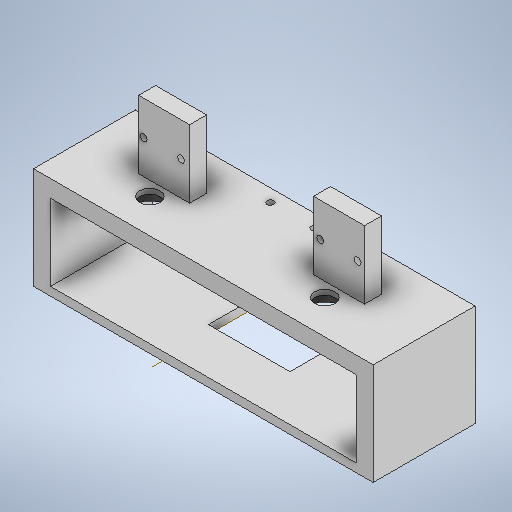
# Autodesk Inventor part: upper part shooter
Saved by Autodesk Inventor 2025.3 (Build 293356000, 356)
## iProperties
Created: 2026-04-10
Part Number: upper part shooter
Material: Generic
Document SubType Name: Modeling
Designer: lenovo
Density: 1 g/cm^3
Appearance: Default
Author: lenovo
## iProperties of the stored document upper part shooter_3DPrint.ipt
Created: 2026-04-14
Part Number: upper part shooter_3DPrint
Material: Generic
Document SubType Name: Modeling
Designer: lenovo
Density: 1 g/cm^3
Appearance: Default
Author: lenovo
Autodesk Inventor part; units mm, degrees
ref_plane "YZ Plane" through (0, 0, 0) normal (1, 0, 0) x (0, 1, 0)
ref_plane "XZ Plane" through (0, 0, 0) normal (0, 1, 0) x (-1, 0, 0)
ref_plane "XY Plane" through (0, 0, 0) normal (0, 0, 1) x (1, 0, 0)
sketch "Sketch1" plane through (0, 0, 0) normal (0, 1, 0) x (-1, 0, 0)
  line L0 (0, -35) -> (4, -35)
  line L1 (-48, 0) -> (-48, -35)
  line L2 (-48, -24.7754) -> (-48, -13.3333)
  line L3 (-48, -35) -> (-52, -35)
  line L4 (-52, -35) -> (-52, -33)
  line L5 (-52, -33) -> (-124, -33)
  line L6 (4, -35) -> (4, -33)
  line L7 (4, -33) -> (76, -33)
  line L8 (0, 0) -> (0, -35)
  line L9 (0, -96.6) -> (0, 47.6) projected
  line L10 (0, 0) -> (-48, 0)
  line L11 (76, -33) -> (76, 27)
  line L12 (76, 27) -> (-124, 27)
  line L13 (-124, 27) -> (-124, -33)
  line L14 (-24, 27) -> (-24, -76) construction
  dimension "d0" = 35
  dimension "d1" = 35
  dimension "d3" = 4
  dimension "d4" = 2
  dimension "d6" = 48
  dimension "d13" = 60
  dimension "d20" = 100
  constraints: 28 end point, 5 perpendicular, 5 vertical, 3 equal length, 3 horizontal, 1 midpoint, 1 parallel, 1 vertical alignment
  measures "d0" distance of L8.start L0.start
  measures "d1" distance of L1.start L1.end
  measures "d3" distance of L1.end L3.end
  measures "d4" distance of L3.end L4.end
  measures "d6" distance of L8.start L1.start
  measures "d13" distance of L7.end L11.end
  measures "d20" distance between parallel lines of L14 L11
extrude "Extrusion1" add sketch "Sketch1" along normal blind 5
sketch "Sketch2" plane through (0, 5, 0) normal (0, 1, 0) x (1, 0, 0)
  line L0 (-4, 35) -> (-4, 33) projected
  line L1 (0, 0) -> (0, 35) projected
  line L2 (-4, 35) -> (0, 35)
  line L3 (0, 35) -> (0, 25)
  line L4 (0, 25) -> (-4, 25)
  line L5 (-4, 25) -> (-4, 35)
  line L6 (52, 35) -> (48, 35) projected
  line L7 (52, 35) -> (48, 35)
  line L8 (48, 35) -> (48, 25)
  line L9 (48, 25) -> (52, 25)
  line L10 (52, 25) -> (52, 35)
  dimension "d21" = 10
  dimension "d22" = 10
  constraints: 16 end point, 4 parallel, 2 horizontal, 2 perpendicular, 1 point on line
  measures "d21" distance of L2.end L3.end
  measures "d22" distance of L8.end L7.end
extrude "Extrusion2" add sketch "Sketch2" along normal blind 10
sketch "Sketch3" plane through (-4, 0, -35) normal (-1, 0, 0) x (0, 0, 1)
  circle A0 centre (5, 10) radius 2
  line L0 (0, 0) -> (0, 15) projected
  line L1 (0, 15) -> (10, 15) projected
  point P0 (35, 0)
  dimension "d25" = 4
  dimension "d26" = 5
  dimension "d27" = 5
  constraints: 1 centre point
  measures "d25" diameter of A0
  measures "d26" distance from line of L0 A0.centre
  measures "d27" distance from line of L1 A0.centre
extrude "Extrusion3" cut sketch "Sketch3" against normal through all
sketch "Sketch7" plane through (0, 5, 0) normal (0, 1, 0) x (1, 0, 0)
  line L0 (-4, 33) -> (-76, 33) projected
  line L1 (-76, -27) -> (124, -27) projected
  line L2 (-76, 33) -> (-66, 33)
  line L3 (-66, 33) -> (-66, -27)
  line L4 (-66, -27) -> (-76, -27)
  line L5 (-76, -27) -> (-76, 33)
  line L6 (124, 33) -> (114, 33)
  line L7 (114, 33) -> (114, -27)
  line L8 (114, -27) -> (124, -27)
  line L9 (124, -27) -> (124, 33)
  point P0 (0, 0)
  dimension "d42" = 10
  dimension "d43" = 10
  dimension "d67" = 190
  constraints: 16 end point, 4 parallel, 3 point on line, 2 horizontal, 2 perpendicular
  measures "d42" distance of L3.end L4.end
  measures "d43" distance of L8.end L7.end
  measures "d67" distance between parallel lines of L7 L5
extrude "Extrusion7" add sketch "Sketch7" along normal blind 45
sketch "Sketch8" plane through (0, 50, 0) normal (0, 1, 0) x (1, 0, 0)
  line L0 (-76, -27) -> (-76, 33)
  line L1 (124, -27) -> (124, 33) projected
  line L2 (-76, -27) -> (124, -27)
  line L3 (124, -27) -> (124, 33)
  line L4 (124, 33) -> (-76, 33)
  line L5 (-76, 33) -> (-76, -27)
  constraints: 10 end point, 2 parallel, 1 horizontal, 1 perpendicular
extrude "Extrusion8" add sketch "Sketch8" along normal blind 10
sketch "Sketch9" plane through (0, 50, 0) normal (0, -1, 0) x (1, 0, 0)
  line L0 (48, -35) -> (48, -25) projected
  line L1 (0, 0) -> (0, -35) projected
  line L2 (0, -33) -> (48, -33)
  line L3 (48, -33) -> (48, -18)
  line L4 (48, -18) -> (0, -18)
  line L5 (0, -18) -> (0, -33)
  dimension "d50" = 15
  constraints: 8 end point, 2 parallel, 2 point on line, 1 horizontal, 1 perpendicular
  measures "d50" distance of L3.end L2.end
extrude "Extrusion9" cut sketch "Sketch9" against normal blind 2.5
sketch "Sketch10" plane through (0, 52.5, 0) normal (0, -1, 0) x (1, 0, 0)
  line L0 (0, -25.5) -> (11, -25.5)
  line L1 (0, 0) -> (0, -35) projected
  circle A0 centre (11, -25.5) radius 2
  line L2 (48, -18) -> (48, -33) projected
  line L3 (48, -25.5) -> (37, -25.5)
  circle A1 centre (37, -25.5) radius 2
  line L4 (48, -33) -> (0, -33) projected
  dimension "d55" = 11
  dimension "d57" = 4
  dimension "d58" = 11
  dimension "d68" = 7.5
  constraints: 4 end point, 2 centre point, 2 coincident, 2 horizontal, 1 equal radius, 1 midpoint, 1 perpendicular, 1 point on line
  measures "d55" distance of L0.start L0.end
  measures "d57" diameter of A0
  measures "d58" distance of L3.start L3.end
  measures "d68" distance from line of L4 L0.end
extrude "Extrusion10" cut sketch "Sketch10" against normal through all
sketch "Sketch12" plane through (0, 50, 0) normal (0, -1, 0) x (1, 0, 0)
  circle A0 centre (-27.5, 7) radius 10.95
  circle A1 centre (75.5, 7) radius 10.95
  point P0 (0, 0)
  dimension "d64" = 21.9
  constraints: 2 centre point, 2 coincident, 1 equal radius
  measures "d64" diameter of A1
extrude "Extrusion12" cut sketch "Sketch12" against normal blind 7
sketch "Sketch16" plane through (-27.5, 57, 7) normal (0, -1, 0) x (1, 0, 0)
  circle A0 centre (0, 0) radius 6
  circle A1 centre (103, 0) radius 10.95 projected
  circle A2 centre (103, 0) radius 6
  point P0 (27.5, -7)
  dimension "d88" = 12
  constraints: 2 centre point, 1 coincident, 1 equal radius
  measures "d88" diameter of A2
extrude "Extrusion15" cut sketch "Sketch16" against normal through all contours A0 | A2
sketch "Sketch17" plane through (0, 60, 0) normal (0, 1, 0) x (1, 0, 0)
  circle A0 centre (75.5, -7) radius 6 projected
  line L0 (75.5, -7) -> (75.5, 1.4)
  line L1 (60.5, 1.4) -> (90.5, 1.4)
  line L2 (90.5, 1.4) -> (90.5, 11.4)
  line L3 (90.5, 11.4) -> (60.5, 11.4)
  line L4 (60.5, 11.4) -> (60.5, 1.4)
  circle A1 centre (75.5, -7) radius 10.95 projected
  circle A2 centre (-27.5, -7) radius 6 projected
  line L5 (75.5, -7) -> (-27.5, -7)
  line L6 (24, -7) -> (24, -1)
  line L7 (-12.5, 1.4) -> (-42.5, 1.4)
  line L8 (-42.5, 1.4) -> (-42.5, 11.4)
  line L9 (-42.5, 11.4) -> (-12.5, 11.4)
  line L10 (-12.5, 11.4) -> (-12.5, 1.4)
  point P0 (0, 0)
  dimension "d91" = 8.4
  dimension "d92" = 30
  dimension "d93" = 10
  constraints: 22 end point, 4 symmetric about line, 3 vertical, 2 horizontal, 2 midpoint, 2 perpendicular
  measures "d91" distance of L0.start L0.end
  measures "d92" distance of L1.start L1.end
  measures "d93" distance of L1.end L2.end
extrude "Extrusion16" add sketch "Sketch17" along normal blind 40 contours L1 A1 | L1 L4 L3 L2 A1 | L7 L8 L9 L10
sketch "Sketch18" plane through (60.5, 60, -1.4) normal (0, 0, 1) x (1, 0, 0)
  circle A0 centre (4, 20) radius 2
  line L0 (-136.5, 0) -> (63.5, 0) projected
  line L1 (0, 0) -> (0, 40) projected
  line L2 (0, 0) -> (30, 0)
  line L3 (15, 0) -> (15, 6)
  circle A1 centre (26, 20) radius 2
  point P0 (-60.5, -60)
  dimension "d96" = 20
  dimension "d97" = 4
  dimension "d98" = 4
  constraints: 4 end point, 2 centre point, 1 midpoint, 1 point on line, 1 symmetric about line, 1 vertical, 1 other
  measures "d96" distance from line of L0 A0.centre
  measures "d97" diameter of A0
  measures "d98" distance from line of L1 A0.centre
extrude "Extrusion17" cut sketch "Sketch18" against normal through all
sketch "Sketch19" plane through (-42.5, 60, -1.4) normal (0, 0, 1) x (1, 0, 0)
  line L0 (-33.5, 0) -> (166.5, 0) projected
  line L1 (133, 0) -> (-1, 0)
  line L2 (66, 0) -> (66, 10)
  circle A0 centre (107, 20) radius 2 projected
  circle A1 centre (107, 20) radius 2
  circle A2 centre (129, 20) radius 2 projected
  circle A3 centre (129, 20) radius 2
  circle A4 centre (25, 20) radius 2
  circle A5 centre (3, 20) radius 2
  point P0 (42.5, -60)
  constraints: 4 centre point, 4 end point, 2 coincident, 2 point on line, 2 symmetric about line, 1 midpoint, 1 vertical, 2 other
extrude "Extrusion18" cut sketch "Sketch19" against normal through all contours A4 | A5
equation "\"d1\" = d0"
body "Solid1"
